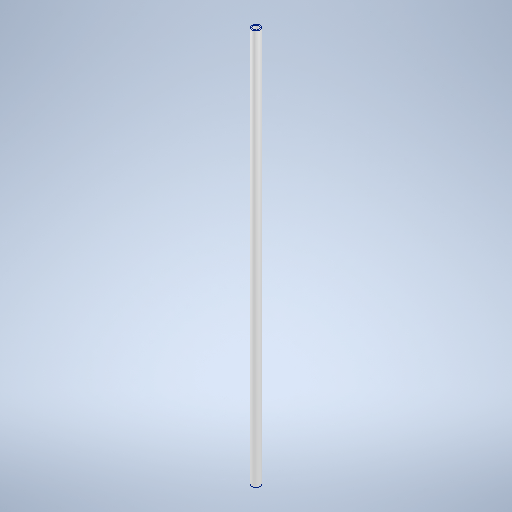
# Autodesk Inventor part: y_rod
Saved by Autodesk Inventor 2025 (Build 290162000, 162)
## iProperties
Created: 2024-04-25
Part Number: y_rod
Material: Hliník 6061
Document SubType Name: Modeling
Designer: rader
Density: 2.7 g/cm^3
Appearance: Hliník – plochý
Author: rader
Autodesk Inventor part; units mm, degrees
ref_plane "YZ Plane" through (0, 0, 0) normal (1, 0, 0) x (0, 1, 0)
ref_plane "XZ Plane" through (0, 0, 0) normal (0, 1, 0) x (-1, 0, 0)
ref_plane "XY Plane" through (0, 0, 0) normal (0, 0, 1) x (1, 0, 0)
sketch "Náčrt1" plane through (0, 0, 0) normal (0, 0, 1) x (1, 0, 0)
  circle A0 centre (0, 0) radius 4
  circle A1 centre (0, 0) radius 3
  dimension "d0" = 8
  dimension "d1" = 6
  constraints: 2 centre point, 2 coincident
  measures "d0" diameter of A0
  measures "d1" diameter of A1
extrude "Vysunutí1" add sketch "Náčrt1" along normal mid plane 387
